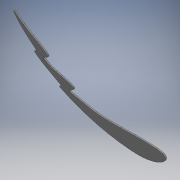
# Autodesk Inventor part: bracket2
Saved by Autodesk Inventor 2018.2 (Build 222227000, 227)
## iProperties
Created: 2018-03-05
Part Number: bracket2
Material: 木材 (オーク)
Document SubType Name: Modeling
Designer: ku_sk
Density: 0.76 g/cm^3
Appearance: ホワイト オーク材 - ナチュラル 標準の光沢
Author: ku_sk
Autodesk Inventor part; units mm, degrees
ref_plane "YZ Plane" through (0, 0, 0) normal (1, 0, 0) x (0, 1, 0)
ref_plane "XZ Plane" through (0, 0, 0) normal (0, 1, 0) x (-1, 0, 0)
ref_plane "XY Plane" through (0, 0, 0) normal (0, 0, 1) x (1, 0, 0)
sketch "スケッチ1" plane through (0, 0, 0) normal (0, 1, 0) x (-1, 0, 0)
  arc A0 (317.1725, 195.8128) -> (314.2512, 198.5108) centre (315.5653, 197.0031) ccw projected
  arc A1 (259.4316, 139.5569) -> (317.1725, 195.8128) centre (115.0525, 345.5076) ccw projected
  arc A2 (250.4691, 133.6616) -> (259.4316, 139.5569) centre (155.393, 287.9636) ccw projected
  arc A3 (232.176, 125.5508) -> (250.4691, 133.6616) centre (211.4405, 197.0022) ccw projected
  arc A4 (219.6233, 123.8241) -> (232.176, 125.5508) centre (220.0183, 167.4446) ccw projected
  arc A5 (215.1935, 124.6186) -> (219.6233, 123.8241) centre (219.7448, 137.2497) ccw projected
  arc A6 (213.6042, 131.9847) -> (215.1935, 124.6186) centre (216.6995, 128.798) ccw projected
  arc A7 (220.1456, 137.3142) -> (213.6042, 131.9847) centre (247.3645, 97.227) ccw projected
  arc A8 (244.0097, 151.903) -> (220.1456, 137.3142) centre (384.6233, -104.9243) ccw projected
  arc A9 (244.0097, 151.903) -> (259.079, 160.1851) centre (-2315.4987, 4826.7805) ccw projected
  arc A10 (259.079, 160.1851) -> (286.3101, 176.9294) centre (95.2726, 457.0952) ccw projected
  arc A11 (286.3101, 176.9294) -> (314.2512, 198.5108) centre (118.2808, 423.3526) ccw projected
  arc A12 (252.3508, 120.9538) -> (250.2273, 124.316) centre (251.1064, 122.5195) ccw projected
  arc A13 (217.6526, 110.7016) -> (250.2273, 124.316) centre (119.1278, 392.2173) ccw projected
  arc A14 (187.0157, 101.5757) -> (217.6526, 110.7016) centre (105.6368, 430.7651) ccw projected
  arc A15 (170.3162, 97.476) -> (187.0157, 101.5757) centre (-1092.0317, 5275.5105) ccw projected
  arc A16 (170.3162, 97.476) -> (143.4895, 89.5609) centre (239.6668, -186.9935) ccw projected
  arc A17 (143.4895, 89.5609) -> (135.7916, 86.106) centre (159.4055, 43.7948) ccw projected
  arc A18 (135.7916, 86.106) -> (135.4203, 78.5795) centre (137.9566, 82.2268) ccw projected
  arc A19 (135.4203, 78.5795) -> (139.4934, 76.6657) centre (143.0857, 89.6023) ccw projected
  arc A20 (139.4934, 76.6657) -> (152.0654, 75.0846) centre (151.1648, 118.6976) ccw projected
  arc A21 (152.0654, 75.0846) -> (171.8343, 78.1844) centre (150.5294, 149.4681) ccw projected
  arc A22 (171.8343, 78.1844) -> (182.0173, 81.5592) centre (119.9342, 251.8363) ccw projected
  arc A23 (182.0173, 81.5592) -> (252.3508, 120.9538) centre (95.8618, 317.8604) ccw projected
  arc A24 (174.7503, 65.8482) -> (173.4237, 69.5954) centre (173.8768, 67.6474) ccw projected
  arc A25 (64.7746, 52.985) -> (173.4237, 69.5954) centre (11.2401, 766.801) ccw projected
  arc A26 (-11.9173, 50.8598) -> (64.7746, 52.985) centre (3.9096, 864.5436) ccw projected
  arc A27 (-53.1769, 51.7289) -> (-11.9173, 50.8598) centre (236.8377, 12839.6895) ccw projected
  arc A28 (-53.1769, 51.7289) -> (-120.2839, 50.0437) centre (-69.1096, -650.8128) ccw projected
  arc A29 (-120.2839, 50.0437) -> (-140.2753, 46.8162) centre (-111.8153, -65.9388) ccw projected
  arc A30 (-140.2753, 46.8162) -> (-145.8114, 29.5987) centre (-137.666, 36.4784) ccw projected
  arc A31 (-145.8114, 29.5987) -> (-137.5577, 22.6319) centre (-121.1943, 50.3906) ccw projected
  arc A32 (-137.5577, 22.6319) -> (-109.3953, 11.1574) centre (-84.3921, 112.8213) ccw projected
  arc A33 (-109.3953, 11.1574) -> (-61.641, 6.0637) centre (-66.7514, 184.549) ccw projected
  arc A34 (-61.641, 6.0637) -> (-35.9382, 7.5619) centre (-74.0904, 440.8658) ccw projected
  arc A35 (-35.9382, 7.5619) -> (174.7503, 65.8482) centre (-88.8837, 608.8772) ccw projected
  line L0 (244.0097, 125.5508) -> (251.3885, 124.4995)
  line L1 (215.1935, 124.6186) -> (228.5578, 119.8031)
  line L2 (228.5578, 119.8031) -> (203.0926, 105.9721)
  line L3 (216.5642, 97.1979) -> (170.3162, 71.9002)
  line L4 (170.3162, 71.9002) -> (174.8442, 69.3979)
  line L5 (136.0222, 78.1844) -> (149.4052, 69.4519)
  line L6 (149.4052, 69.4519) -> (64.7767, 52.9852)
  line L7 (244.0097, 125.5508) -> (276.1369, 152.3423)
  point P0 (0, 0)
  constraints: 16 end point, 7 point on circle, 6 tangent
extrude "押し出し1" add sketch "スケッチ1" along normal blind 4
fillet "フィレット1" radius 2 4 edges at (-228.5578, 2, 119.8031) (-149.4052, 2, 69.4519) (-244.0097, 2, 125.5508) (-170.3162, 2, 71.9002)
fillet "フィレット1" radius 30 2 edges at (-203.0926, 2, 105.9721) (-64.7767, 2, 52.9852)
